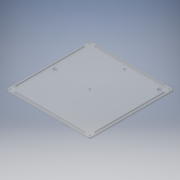
# Autodesk Inventor part: Main
Saved by Autodesk Inventor 2016 (Build 200138000, 138)
## iProperties
Created: 2018-04-27
Part Number: Main
Material: Polycarbonate, Clear
Document SubType Name: Modeling
Designer: Phil Erle
Density: 1.2 g/cm^3
Appearance: Polycarbonate - Clear
Author: Phil Erle
Autodesk Inventor part; units mm, degrees
ref_plane "YZ Plane" through (0, 0, 0) normal (1, 0, 0) x (0, 1, 0)
ref_plane "XZ Plane" through (0, 0, 0) normal (0, 1, 0) x (-1, 0, 0)
ref_plane "XY Plane" through (0, 0, 0) normal (0, 0, 1) x (1, 0, 0)
sketch "Sketch1" plane through (0, 0, 0) normal (0, 0, 1) x (1, 0, 0)
  line L0 (-145, -145) -> (145, -145)
  line L1 (145, -145) -> (145, 145)
  line L2 (145, 145) -> (-145, 145)
  line L3 (-145, 145) -> (-145, -145)
  line L4 (-145, -145) -> (145, 145) construction
  line L5 (145, -145) -> (-145, 145) construction
  point P0 (0, 0)
  dimension "d0" = 290
  dimension "d1" = 290
  constraints: 12 end point, 2 midpoint, 2 parallel, 1 horizontal, 1 perpendicular
  measures "d0" distance of L2.end L1.end
  measures "d1" distance of L1.end L0.end
extrude "Extrusion1" add sketch "Sketch1" along normal blind 5
sketch "Sketch2" plane through (0, 0, 5) normal (0, 0, 1) x (1, 0, 0)
  point P0 (0, 0)
  point P1 (0, 0)
  constraints: 1 coincident
hole "Hole1" at (0, 0, 5) direction (0, 0, -1) diameter 6.6 depth 8 tip angle 118 clearance for "Countersunk Flat Head Screw DIN EN ISO 2009" size "M6" standard "DIN"
sketch "Sketch3" plane through (0, 0, 5) normal (0, 0, 1) x (1, 0, 0)
  line L0 (-137.5, -137.5) -> (137.5, -137.5) construction
  line L1 (137.5, -137.5) -> (137.5, 137.5) construction
  line L2 (137.5, 137.5) -> (-137.5, 137.5) construction
  line L3 (-137.5, 137.5) -> (-137.5, -137.5) construction
  line L4 (-137.5, -137.5) -> (137.5, 137.5) construction
  line L5 (137.5, -137.5) -> (-137.5, 137.5) construction
  point P0 (0, 0)
  dimension "d11" = 275
  dimension "d12" = 275
  constraints: 12 end point, 4 coincident, 2 midpoint, 2 parallel, 1 horizontal, 1 perpendicular
  measures "d11" distance of L2.end L1.end
  measures "d12" distance of L1.end L0.end
hole "Hole2" at (-137.5, 137.5, 5) at (137.5, 137.5, 5) at (137.5, -137.5, 5) at (-137.5, -137.5, 5) direction (0, 0, -1) diameter 5.5 depth 8 tip angle 118 clearance for "Countersunk Flat Head Screw DIN EN ISO 2009" size "M5" standard "DIN"
fillet "Fillet1" radius 6 4 edges at (-145, -145, 2.5) (145, -145, 2.5) (145, 145, 2.5) (-145, 145, 2.5)
sketch "Sketch4" plane through (0, 0, 5) normal (0, 0, 1) x (1, 0, 0)
  line L0 (-120, -140) -> (120, -140)
  line L1 (120, -140) -> (120, -135)
  line L2 (120, -135) -> (-120, -135)
  line L3 (-120, -135) -> (-120, -140)
  line L4 (140, -120) -> (135, -120)
  line L5 (135, -120) -> (135, 120)
  line L6 (135, 120) -> (140, 120)
  line L7 (140, 120) -> (140, -120)
  line L8 (120, 141) -> (-120, 141)
  line L9 (-120, 141) -> (-120, 136)
  line L10 (-120, 136) -> (120, 136)
  line L11 (120, 136) -> (120, 141)
  line L12 (-135, 120) -> (-140, 120)
  line L13 (-140, 120) -> (-140, -120)
  line L14 (-140, -120) -> (-135, -120)
  line L15 (-135, -120) -> (-135, 120)
  line L16 (-139, -145) -> (139, -145) projected
  line L17 (145, -139) -> (145, 139) projected
  line L18 (139, 145) -> (-139, 145) projected
  line L19 (-145, 139) -> (-145, -139) projected
  point P0 (0, 0)
  point P1 (0, 136)
  point P2 (-135, 0)
  dimension "d21" = 5
  dimension "d22" = 5
  dimension "d23" = 240
  dimension "d24" = 240
  dimension "d25" = 5
  dimension "d26" = 5
  dimension "d27" = 5
  dimension "d28" = 5
  dimension "d29" = 4
  dimension "d30" = 5
  constraints: 32 end point, 8 parallel, 4 horizontal, 4 perpendicular, 4 point on line, 2 midpoint, 1 horizontal alignment, 1 vertical alignment
  measures "d21" distance of L12.start L12.end
  measures "d22" distance of L8.end L9.end
  measures "d23" distance of L12.end L13.end
  measures "d24" distance of L8.start L8.end
  measures "d25" distance of L2.end L0.start
  measures "d26" distance of L4.start L4.end
  measures "d27" distance between parallel lines of L19 L13
  measures "d28" distance between parallel lines of L16 L0
  measures "d29" distance between parallel lines of L18 L8
  measures "d30" distance between parallel lines of L17 L7
extrude "Extrusion2" cut sketch "Sketch4" against normal through all
sketch "Sketch5" plane through (0, 0, 5) normal (0, 0, 1) x (1, 0, 0)
  point P0 (0, 0)
  point P1 (-120, 0)
  point P2 (120, 120)
  dimension "d34" = 120
  dimension "d51" = 120
  dimension "d52" = 120
  constraints: 1 horizontal alignment
  measures "d34" distance of point (0, 0) point (-120, 0)
  measures "d51" horizontal distance of point (120, 120) point (0, 0)
  measures "d52" horizontal distance of point (0, 0) point (120, 120)
hole "Hole3" at (-120, 0, 5) at (120, 120, 5) direction (0, 0, -1) diameter 12 depth 8 tip angle 118
sketch "Sketch6" plane through (0, 0, 5) normal (0, 0, 1) x (1, 0, 0)
  point P0 (0, 0)
  point P1 (0, 120)
  dimension "d50" = 120
  constraints: 1 vertical alignment
  measures "d50" distance of point (0, 120) point (0, 0)
hole "Hole4" at (0, 120, 5) direction (0, 0, -1) diameter 8 depth 8 tip angle 118
body "Solid1"
